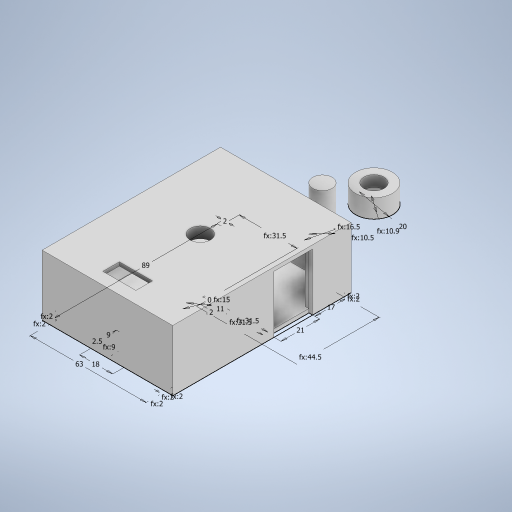
# Autodesk Inventor part: REceiver
Saved by Autodesk Inventor 2024 (Build 280153000, 153)
## iProperties
Created: 2023-11-02
Part Number: REceiver
Material: Generic
Document SubType Name: Modeling
Designer: Lukas
Density: 1 g/cm^3
Appearance: Default
Author: Lukas
Autodesk Inventor part; units mm, degrees
ref_plane "YZ Plane" through (0, 0, 0) normal (1, 0, 0) x (0, 1, 0)
ref_plane "XZ Plane" through (0, 0, 0) normal (0, 1, 0) x (-1, 0, 0)
ref_plane "XY Plane" through (0, 0, 0) normal (0, 0, 1) x (1, 0, 0)
sketch "Bottom_sketch" plane through (0, 0, 0) normal (0, 1, 0) x (-1, 0, 0)
  line L0 (31.5, 44.5) -> (-31.5, 44.5)
  line L1 (-31.5, 44.5) -> (-31.5, -44.5)
  line L2 (-31.5, -44.5) -> (31.5, -44.5)
  line L3 (31.5, -44.5) -> (31.5, 44.5)
  line L4 (31.5, 44.5) -> (33.5, 44.5)
  line L5 (33.5, 44.5) -> (33.5, -44.5)
  line L6 (33.5, -44.5) -> (31.5, -44.5)
  line L7 (31.5, -44.5) -> (31.5, 44.5)
  line L8 (-31.5, 44.5) -> (-33.5, 44.5)
  line L9 (-33.5, 44.5) -> (-33.5, -44.5)
  line L10 (-33.5, -44.5) -> (-31.5, -44.5)
  line L11 (-31.5, -44.5) -> (-31.5, 44.5)
  line L12 (33.5, 44.5) -> (-33.5, 44.5)
  line L13 (-33.5, 44.5) -> (-33.5, 46.5)
  line L14 (-33.5, 46.5) -> (33.5, 46.5)
  line L15 (33.5, 46.5) -> (33.5, 44.5)
  line L16 (33.5, -44.5) -> (-33.5, -44.5)
  line L17 (-33.5, -44.5) -> (-33.5, -46.5)
  line L18 (-33.5, -46.5) -> (33.5, -46.5)
  line L19 (33.5, -46.5) -> (33.5, -44.5)
  line L20 (33.5, 46.5) -> (35.5, 46.5)
  line L21 (35.5, 46.5) -> (35.5, -46.5)
  line L22 (35.5, -46.5) -> (33.5, -46.5)
  line L23 (33.5, -46.5) -> (33.5, 46.5)
  line L24 (-33.5, 46.5) -> (-35.5, 46.5)
  line L25 (-35.5, 46.5) -> (-35.5, -46.5)
  line L26 (-35.5, -46.5) -> (-33.5, -46.5)
  line L27 (-33.5, -46.5) -> (-33.5, 46.5)
  line L28 (35.5, 46.5) -> (-35.5, 46.5)
  line L29 (-35.5, 46.5) -> (-35.5, 48.5)
  line L30 (-35.5, 48.5) -> (35.5, 48.5)
  line L31 (35.5, 48.5) -> (35.5, 46.5)
  line L32 (35.5, -46.5) -> (-35.5, -46.5)
  line L33 (-35.5, -46.5) -> (-35.5, -48.5)
  line L34 (-35.5, -48.5) -> (35.5, -48.5)
  line L35 (35.5, -48.5) -> (35.5, -46.5)
  line L36 (-31.5, -27.5) -> (-35.5, -27.5)
  line L37 (-35.5, -27.5) -> (-35.5, -6.5)
  line L38 (-35.5, -6.5) -> (-31.5, -6.5)
  line L39 (-31.5, -6.5) -> (-31.5, -27.5)
  line L40 (9, 48.5) -> (-9, 48.5)
  line L41 (-9, 48.5) -> (-9, 44.5)
  line L42 (-9, 44.5) -> (9, 44.5)
  line L43 (9, 44.5) -> (9, 48.5)
  circle A0 centre (0, -2) radius 5.5
  circle A1 centre (0, -2) radius 7.5
  line L44 (9, 42) -> (-9, 42)
  line L45 (-9, 42) -> (-9, 33)
  line L46 (-9, 33) -> (9, 33)
  line L47 (9, 33) -> (9, 42)
  circle A2 centre (0, -68.419) radius 5.25
  circle A3 centre (0, -68.419) radius 8.25
  circle A4 centre (0, -96.4402) radius 10
  circle A5 centre (0, -96.4402) radius 5.45
  point P0 (0, 0)
  point P1 (-33.5, -44.5)
  point P2 (-31.5, -6.5)
  point P3 (-33.5, -6.5)
  point P4 (-33.5, -27.5)
  point P5 (-31.5, -27.5)
  point P6 (-35.5, -27.5)
  point P7 (0, 46.5)
  point P8 (-9, 48.5)
  point P9 (-9, 44.5)
  point P10 (9, 46.5)
  point P11 (-9, 46.5)
  dimension "width" = 89
  dimension "height" = 63
  dimension "d6" = 31.5
  dimension "d7" = 44.5
  dimension "thickness" = 2
  dimension "d9" = 2
  dimension "d10" = 2
  dimension "d11" = 2
  dimension "d16" = 2
  dimension "d17" = 2
  dimension "d18" = 2
  dimension "d19" = 2
  dimension "lora_width" = 21
  dimension "d25" = 17
  dimension "d28" = 18
  dimension "d29" = 9
  dimension "d39" = 2
  dimension "d40" = 11
  dimension "d42" = 15
  dimension "d45" = 2.5
  dimension "d46" = 9
  dimension "d49" = 10.5
  dimension "d53" = 31.5
  dimension "d54" = 31.5
  dimension "d55" = 0
  dimension "d56" = 16.5
  dimension "d59" = 20
  dimension "d62" = 10.9
  constraints: 96 end point, 24 parallel, 12 horizontal, 12 perpendicular, 7 collinear, 7 point on line, 6 centre point, 2 coincident, 1 midpoint, 2 other
  measures "width" distance between parallel lines of L2 L0
  measures "height" distance between parallel lines of L3 L1
  measures "d6" distance from line of point (0, 0) L3
  measures "d7" distance from line of L2 point (0, 0)
  measures "thickness" distance of L5.end L6.end
  measures "d9" distance between parallel lines of L0 L14
  measures "d10" distance between parallel lines of L1 L9
  measures "d11" distance between parallel lines of L16 L18
  measures "d16" distance between parallel lines of L5 L21
  measures "d17" distance between parallel lines of L9 L25
  measures "d18" distance between parallel lines of L28 L30
  measures "d19" distance between parallel lines of L32 L34
  measures "lora_width" distance between parallel lines of L36 L38
  measures "d25" distance between parallel lines of L2 L36
  measures "d28" distance between parallel lines of L41 L43
  measures "d29" distance from line of point (0, 46.5) L43
  measures "d39" distance of point (0, 0) A0.centre
  measures "d40" diameter of A0
  measures "d42" diameter of A1
  measures "d45" distance between parallel lines of L44 L0
  measures "d46" distance between parallel lines of L46 L44
  measures "d49" diameter of A2
  measures "d53" distance from line of L1 A0.centre
  measures "d54" distance from line of L1 A1.centre
  measures "d55" distance of A1.centre A0.centre
  measures "d56" diameter of A3
  measures "d59" diameter of A4
  measures "d62" diameter of A5
extrude "Bottom" add sketch "Bottom_sketch" along normal blind 2 contours L3 L2 L1 L0 | A0 | A1 | L47 L46 L45 L44
extrude "Side_Inside" add sketch "Bottom_sketch" along normal blind 30 contours L4 L5 L6 L3 | L0 L43 L14 L15 L4 | L0 L41 L14 L43 | L6 L19 L18 L17 L10 L2 | L0 L8 L13 L14 L41 | L10 L9 L36 L1 | L1 L38 L9 L8 | L36 L9 L38 L1
extrude "Side_Outside" add sketch "Bottom_sketch" along normal blind 31 separate body contours L15 L20 L21 L22 L19 L5 | L43 L30 L31 L20 L14 | L14 L41 L30 L43 | L14 L24 L29 L30 L41 | L17 L26 L25 L36 L9 | L22 L35 L34 L33 L26 L18 | L9 L38 L25 L24 L13 | L36 L25 L38 L9
extrude "Top" add sketch "Bottom_sketch" along normal blind 2 from surface at 31 contours L3 L2 L1 L0 | L4 L5 L6 L3 | L0 L43 L14 L15 L4 | L0 L41 L14 L43 | L6 L19 L18 L17 L10 L2 | L15 L20 L21 L22 L19 L5 | L0 L8 L13 L14 L41 | L43 L30 L31 L20 L14 | L14 L41 L30 L43 | L10 L9 L36 L1 | L1 L38 L9 L8 | L14 L24 L29 L30 L41 | L36 L9 L38 L1 | L17 L26 L25 L36 L9 | L22 L35 L34 L33 L26 L18 | L9 L38 L25 L24 L13 | L36 L25 L38 L9 | A0 | A1 | L47 L46 L45 L44 bodies 2
extrude "Lora_Hole" cut sketch "Bottom_sketch" along normal blind 29 from surface at 2 contours L36 L9 L38 L1 | L36 L25 L38 L9 bodies 1 2
extrude "TTL_Hole" [suppressed]
extrude "TTL_Outside" [suppressed]
extrude "Button_Hole" cut sketch "Bottom_sketch" against normal blind 6 from surface at 33 contours A0 bodies 1 2
extrude "Lora_Outside" cut sketch "Bottom_sketch" along normal blind 3 contours L36 L25 L38 L9 bodies 1 2
extrude "Button_slide" add sketch "Bottom_sketch" against normal blind 4 from surface at 31 contours A1 bodies 2
extrude "TTL_Hole_v2" cut sketch "Bottom_sketch" along normal blind 6 from surface at 31 contours L47 L46 L45 L44 bodies 2
extrude "Button_Piece" add sketch "Bottom_sketch" along normal blind 24 separate body contours A2
extrude "Button_Bottom" add sketch "Bottom_sketch" along normal blind 3 contours A3 bodies 3
extrude "Button_Mushroom" add sketch "Bottom_sketch" along normal blind 10 contours A4 | A5 bodies 3
extrude "Mushroom_Inside" cut sketch "Bottom_sketch" against normal blind 6 from surface at 10 contours A5 bodies 3
equation "\"d6\" = 0.5 * height"
equation "\"d7\" = 0.5 * width"
equation "\"d9\" = thickness"
equation "\"d10\" = thickness"
equation "\"d11\" = thickness"
equation "\"d16\" = thickness"
equation "\"d17\" = thickness"
equation "\"d18\" = thickness"
equation "\"d19\" = thickness"
equation "\"d29\" = 0.5 * d28"
equation "\"d42\" = d40 + 2 * thickness"
equation "\"d53\" = 0.5 * height"
equation "\"d54\" = d53"
equation "\"d12\" = thickness"
equation "\"d22\" = thickness"
equation "\"d30\" = depth - 1.5 * thickness"
equation "\"d35\" = 1.5 * thickness"
equation "\"d33\" = 3 * thickness"
equation "\"d37\" = 1.5 * thickness"
equation "\"d47\" = 3 * thickness"
equation "\"d50\" = 0.8 * depth"
equation "\"depth\" = 30"
